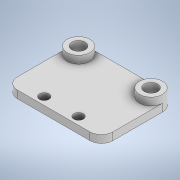
# Autodesk Inventor part: Xenstopmount
Saved by Autodesk Inventor 2020.2 (Build 242310000, 310)
## iProperties
Created: 2020-08-25
Part Number: Xenstopmount
Material: Generic
Document SubType Name: Modeling
Designer: JK
Density: 1 g/cm^3
Appearance: Default
Author: JK
Autodesk Inventor part; units mm, degrees
ref_plane "YZ Plane" through (0, 0, 0) normal (1, 0, 0) x (0, 1, 0)
ref_plane "XZ Plane" through (0, 0, 0) normal (0, 1, 0) x (-1, 0, 0)
ref_plane "XY Plane" through (0, 0, 0) normal (0, 0, 1) x (1, 0, 0)
sketch "Sketch1" plane through (0, 0, 0) normal (0, 1, 0) x (-1, 0, 0)
  line L0 (-12.5, 12.5) -> (12.5, 12.5)
  line L1 (12.5, 12.5) -> (12.5, -12.5)
  line L2 (12.5, -12.5) -> (-12.5, -12.5)
  line L3 (-12.5, -12.5) -> (-12.5, 12.5)
  line L4 (-12.5, 12.5) -> (12.5, -12.5) construction
  line L5 (12.5, 12.5) -> (-12.5, -12.5) construction
  circle A0 centre (4.5, 4.5) radius 1.25
  circle A1 centre (-4.5, 4.5) radius 1.25
  circle A2 centre (9.5, -9.5) radius 1.75
  circle A3 centre (-9.5, -9.5) radius 1.75
  line L6 (12.5, 12.5) -> (-12.5, 12.5)
  line L7 (-12.5, 12.5) -> (-12.5, 6.5)
  line L8 (-12.5, 6.5) -> (12.5, 6.5)
  line L9 (12.5, 6.5) -> (12.5, 12.5)
  point P0 (0, 0)
  dimension "d0" = 3.5
  dimension "d1" = 19
  dimension "d3" = 3
  dimension "d4" = 3
  dimension "d5" = 3
  dimension "d6" = 9
  dimension "d7" = 14
  dimension "d8" = 2.5
  dimension "d9" = 4.5
  dimension "d10" = 6
  constraints: 20 end point, 4 centre point, 4 parallel, 2 equal radius, 2 horizontal, 2 horizontal alignment, 2 midpoint, 2 perpendicular, 2 point on line
  measures "d0" diameter of A2
  measures "d1" distance of A2.centre A3.centre
  measures "d3" distance from line of L1 A2.centre
  measures "d4" distance from line of L2 A2.centre
  measures "d5" distance from line of L3 A3.centre
  measures "d6" distance of A0.centre A1.centre
  measures "d7" vertical distance of A2.centre A0.centre
  measures "d8" diameter of A0
  measures "d9" horizontal distance of A0.centre point (0, 0)
  measures "d10" distance between parallel lines of L6 L8
extrude "Extrusion1" add sketch "Sketch1" along normal blind 2 contours L8 L1 L2 L3
sketch "Sketch2" plane through (0, 2, 0) normal (0, 1, 0) x (1, 0, 0)
  circle A0 centre (-9.5, 9.5) radius 1.75 projected
  circle A1 centre (-9.5, 9.5) radius 3
  circle A2 centre (9.5, 9.5) radius 1.75 projected
  circle A3 centre (9.5, 9.5) radius 3
  circle A4 centre (-9.5, 9.5) radius 1.75 projected
  circle A5 centre (9.5, 9.5) radius 1.75 projected
  point P0 (0, 0)
  dimension "d13" = 6
  dimension "d14" = 6
  constraints: 2 centre point, 2 coincident
  measures "d13" diameter of A1
  measures "d14" diameter of A3
extrude "Extrusion2" add sketch "Sketch2" along normal blind 2
fillet "Fillet1" radius 3 4 edges at (12.5, 1, -12.5) (12.5, 1, 6.5) (-12.5, 1, -12.5) (-12.5, 1, 6.5)
body "Solid1"
